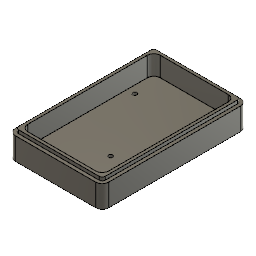
newboxbottom v3 (Autodesk Fusion 360 design; units mm, degrees)
Autodesk Fusion 360 part; units mm, degrees
sketch "Sketch1" plane through (0, 0, 0) normal (0, 1, 0) x (1, 0, 0)
  line L0 (36.83, -57.15) -> (-36.83, -57.15)
  line L1 (-36.83, -57.15) -> (-36.83, 57.15)
  line L2 (-36.83, 57.15) -> (36.83, 57.15)
  line L3 (36.83, 57.15) -> (36.83, -57.15)
  line L4 (36.83, -57.15) -> (-36.83, 57.15) construction
  line L5 (-36.83, -57.15) -> (36.83, 57.15) construction
  dimension "d1" = 73.66
  dimension "d2" = 114.3
extrude "Extrude1" add sketch "Sketch1" along normal blind 20.32
shell "Shell1" thickness 4.953 removed faces 1 at (-12.2767, 20.32, 19.05)
sketch "Sketch2" plane through (0, 4.953, 0) normal (0, 1, 0) x (-1, 0, 0)
  line L0 (-31.877, -52.197) -> (31.877, -52.197)
  line L1 (31.877, -52.197) -> (31.877, 52.197)
  line L2 (31.877, 52.197) -> (-31.877, 52.197)
  line L3 (-31.877, 52.197) -> (-31.877, -52.197)
  circle A0 centre (25.8572, -31.2674) radius 1.6002
  circle A1 centre (-22.4028, -29.9974) radius 1.6002
  circle A2 centre (-7.1628, 20.8026) radius 1.6002
  dimension "d6" = 3.2004
  dimension "d7" = 3.2004
  dimension "d8" = 3.2004
  dimension "d9" = 6.0198
  dimension "d10" = 20.9296
  dimension "d13" = 22.1996
  dimension "d14" = 48.26
  dimension "d15" = 33.02
  dimension "d16" = 52.07
  measures "d6" diameter of A0
  measures "d7" diameter of A1
  measures "d8" diameter of A2
  measures "d15" distance of origin
  measures "d16" distance of origin
extrude "Extrude2" cut sketch "Sketch2" against normal through all contours A0 | A1 | A2
fillet "Fillet1" radius 5.08 4 edges at (-36.83, 10.16, 57.15) (36.83, 10.16, 57.15) (36.83, 10.16, -57.15) (-36.83, 10.16, -57.15)
fillet "Fillet2" radius 5.08 4 edges at (-31.877, 12.6365, -52.197) (-31.877, 12.6365, 52.197) (31.877, 12.6365, 52.197) (31.877, 12.6365, -52.197)
sketch "Sketch3" plane through (0, 20.32, 0) normal (0, 1, 0) x (-1, 0, 0)
  arc A0 (31.75, -57.15) -> (36.83, -52.07) centre (31.75, -52.07) ccw
  line L0 (36.83, -52.07) -> (36.83, 52.07)
  arc A1 (36.83, 52.07) -> (31.75, 57.15) centre (31.75, 52.07) ccw
  line L1 (31.75, 57.15) -> (-31.75, 57.15)
  arc A2 (-31.75, 57.15) -> (-36.83, 52.07) centre (-31.75, 52.07) ccw
  line L2 (-36.83, 52.07) -> (-36.83, -52.07)
  arc A3 (-36.83, -52.07) -> (-31.75, -57.15) centre (-31.75, -52.07) ccw
  line L3 (-31.75, -57.15) -> (31.75, -57.15)
  line L4 (-31.877, -47.117) -> (-31.877, 47.117)
  arc A4 (-26.797, 52.197) -> (-31.877, 47.117) centre (-26.797, 47.117) ccw
  line L5 (-26.797, 52.197) -> (26.797, 52.197)
  arc A5 (31.877, 47.117) -> (26.797, 52.197) centre (26.797, 47.117) ccw
  line L6 (31.877, 47.117) -> (31.877, -47.117)
  arc A6 (26.797, -52.197) -> (31.877, -47.117) centre (26.797, -47.117) ccw
  line L7 (26.797, -52.197) -> (-26.797, -52.197)
  arc A7 (-31.877, -47.117) -> (-26.797, -52.197) centre (-26.797, -47.117) ccw
  line L8 (-31.75, -54.483) -> (31.75, -54.483)
  arc A8 (31.75, -54.483) -> (34.163, -52.07) centre (31.75, -52.07) ccw
  line L9 (34.163, -52.07) -> (34.163, 52.07)
  arc A9 (34.163, 52.07) -> (31.75, 54.483) centre (31.75, 52.07) ccw
  line L10 (31.75, 54.483) -> (-31.75, 54.483)
  arc A10 (-31.75, 54.483) -> (-34.163, 52.07) centre (-31.75, 52.07) ccw
  line L11 (-34.163, 52.07) -> (-34.163, -52.07)
  arc A11 (-34.163, -52.07) -> (-31.75, -54.483) centre (-31.75, -52.07) ccw
  dimension "d20" = 2.667
extrude "Extrude3" cut sketch "Sketch3" against normal blind 2.667 contours A0 L0 A1 L1 A2 L2 A3 L3
